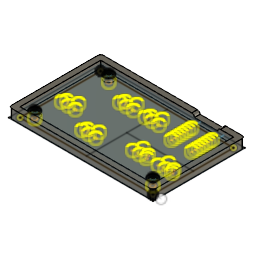
tetriopadv2_assembly (Autodesk Fusion 360 archive; units mm, degrees)
design "tetrio.padv2"
Autodesk Fusion 360 part; units mm, degrees
sketch "Sketch1" plane through (0, 0, -0.05) normal (0, 0, -1) x (1, 0, 0)
  line L0 (69.1388, 132.6388) -> (69.1388, 72.5424)
  line L1 (69.1388, 72.5424) -> (168.3004, 72.5424)
  line L2 (168.3004, 72.5424) -> (168.3004, 132.6388)
  line L3 (168.3004, 132.6388) -> (69.1388, 132.6388)
  circle A0 centre (75.184, 127.762) radius 1.5875
  circle A1 centre (162.6616, 127.1016) radius 1.5875
  circle A2 centre (105.5624, 117.7544) radius 1.9875
  circle A3 centre (100.4824, 117.7544) radius 0.8374
  circle A4 centre (110.6424, 117.7544) radius 0.8374
  circle A5 centre (101.7524, 115.2144) radius 0.7374
  circle A6 centre (137.5664, 111.8616) radius 1.9875
  circle A7 centre (156.6164, 111.8616) radius 1.9875
  circle A8 centre (108.1024, 112.6744) radius 0.7374
  circle A9 centre (132.4864, 111.8616) radius 0.8374
  circle A10 centre (142.6464, 111.8616) radius 0.8374
  circle A11 centre (151.5364, 111.8616) radius 0.8374
  circle A12 centre (161.6964, 111.8616) radius 0.8374
  circle A13 centre (141.3764, 109.3216) radius 0.7374
  circle A14 centre (160.4264, 109.3216) radius 0.7374
  circle A15 centre (79.5528, 106.9848) radius 1.9875
  circle A16 centre (74.4728, 106.9848) radius 0.8374
  circle A17 centre (84.6328, 106.9848) radius 0.8374
  circle A18 centre (135.0264, 106.7816) radius 0.7374
  circle A19 centre (154.0764, 106.7816) radius 0.7374
  circle A20 centre (75.7428, 104.4448) radius 0.7374
  circle A21 centre (82.0928, 101.9048) radius 0.7374
  circle A22 centre (140.0556, 90.7861) radius 0.4319
  circle A23 centre (155.2956, 90.7861) radius 0.4319
  circle A24 centre (140.0556, 88.2461) radius 0.4319
  circle A25 centre (155.2956, 88.2461) radius 0.4319
  circle A26 centre (101.8032, 85.8012) radius 1.9875
  circle A27 centre (120.8532, 85.8012) radius 1.9875
  circle A28 centre (96.7232, 85.8012) radius 0.8374
  circle A29 centre (106.8832, 85.8012) radius 0.8374
  circle A30 centre (115.7732, 85.8012) radius 0.8374
  circle A31 centre (125.9332, 85.8012) radius 0.8374
  circle A32 centre (140.0556, 85.7061) radius 0.4319
  circle A33 centre (155.2956, 85.7061) radius 0.4319
  circle A34 centre (97.9932, 83.2612) radius 0.7374
  circle A35 centre (117.0432, 83.2612) radius 0.7374
  circle A36 centre (140.0556, 83.1661) radius 0.4319
  circle A37 centre (155.2956, 83.1661) radius 0.4319
  circle A38 centre (104.3432, 80.7212) radius 0.7374
  circle A39 centre (123.3932, 80.7212) radius 0.7374
  circle A40 centre (140.0556, 80.6261) radius 0.4319
  circle A41 centre (155.2956, 80.6261) radius 0.4319
  circle A42 centre (140.0556, 78.0861) radius 0.4319
  circle A43 centre (155.2956, 78.0861) radius 0.4319
  circle A44 centre (79.2988, 76.6064) radius 1.5875
  circle A45 centre (140.0556, 75.5461) radius 0.4319
  circle A46 centre (155.2956, 75.5461) radius 0.4319
  circle A47 centre (75.184, 127.762) radius 1.5875
  circle A48 centre (79.2988, 76.6064) radius 1.5875
  circle A49 centre (162.6616, 127.1016) radius 1.5875
  circle A50 centre (162.6616, 127.1016) radius 3.5
  circle A51 centre (79.2988, 76.6064) radius 3.5
  circle A52 centre (75.184, 127.762) radius 3.5
  dimension "d1" = 7
  dimension "d2" = 7
  dimension "d3" = 7
  constraint concentric A0 A47
  constraint concentric A44 A48
  constraint concentric A1 A49
  constraint concentric A49 A50
  constraint concentric A48 A51
  constraint concentric A47 A52
  measures "d1" diameter of A50
  measures "d2" diameter of A51
  measures "d3" diameter of A52
extrude "Extrude1" add sketch "Sketch1" along normal blind 5 contours A50 | A51 | A52 makes body 1 at (72.8681, -125.1378, -3.3833) makes body 2 at (82.7944, -76.4319, -3.3833) makes body 3 at (165.4516, -129.2149, -3.3833)
sketch "Sketch2" plane through (0, 0, -0.05) normal (0, 0, -1) x (1, 0, 0)
sketch "Sketch3" plane through (0, 0, -5.05) normal (0, 0, -1) x (1, 0, 0)
  circle A0 centre (75.184, 127.762) radius 1.5875
  circle A1 centre (75.184, 127.762) radius 3.5
  line L0 (69.1388, 132.6388) -> (69.1388, 72.5424)
  line L1 (69.1388, 72.5424) -> (168.3004, 72.5424)
  line L2 (168.3004, 72.5424) -> (168.3004, 132.6388)
  line L3 (168.3004, 132.6388) -> (69.1388, 132.6388)
  circle A2 centre (75.184, 127.762) radius 1.5875
  circle A3 centre (162.6616, 127.1016) radius 1.5875
  circle A4 centre (105.5624, 117.7544) radius 1.9875
  circle A5 centre (100.4824, 117.7544) radius 0.8374
  circle A6 centre (110.6424, 117.7544) radius 0.8374
  circle A7 centre (101.7524, 115.2144) radius 0.7374
  circle A8 centre (137.5664, 111.8616) radius 1.9875
  circle A9 centre (156.6164, 111.8616) radius 1.9875
  circle A10 centre (108.1024, 112.6744) radius 0.7374
  circle A11 centre (132.4864, 111.8616) radius 0.8374
  circle A12 centre (142.6464, 111.8616) radius 0.8374
  circle A13 centre (151.5364, 111.8616) radius 0.8374
  circle A14 centre (161.6964, 111.8616) radius 0.8374
  circle A15 centre (141.3764, 109.3216) radius 0.7374
  circle A16 centre (160.4264, 109.3216) radius 0.7374
  circle A17 centre (79.5528, 106.9848) radius 1.9875
  circle A18 centre (74.4728, 106.9848) radius 0.8374
  circle A19 centre (84.6328, 106.9848) radius 0.8374
  circle A20 centre (135.0264, 106.7816) radius 0.7374
  circle A21 centre (154.0764, 106.7816) radius 0.7374
  circle A22 centre (75.7428, 104.4448) radius 0.7374
  circle A23 centre (82.0928, 101.9048) radius 0.7374
  circle A24 centre (140.0556, 90.7861) radius 0.4319
  circle A25 centre (155.2956, 90.7861) radius 0.4319
  circle A26 centre (140.0556, 88.2461) radius 0.4319
  circle A27 centre (155.2956, 88.2461) radius 0.4319
  circle A28 centre (101.8032, 85.8012) radius 1.9875
  circle A29 centre (120.8532, 85.8012) radius 1.9875
  circle A30 centre (96.7232, 85.8012) radius 0.8374
  circle A31 centre (106.8832, 85.8012) radius 0.8374
  circle A32 centre (115.7732, 85.8012) radius 0.8374
  circle A33 centre (125.9332, 85.8012) radius 0.8374
  circle A34 centre (140.0556, 85.7061) radius 0.4319
  circle A35 centre (155.2956, 85.7061) radius 0.4319
  circle A36 centre (97.9932, 83.2612) radius 0.7374
  circle A37 centre (117.0432, 83.2612) radius 0.7374
  circle A38 centre (140.0556, 83.1661) radius 0.4319
  circle A39 centre (155.2956, 83.1661) radius 0.4319
  circle A40 centre (104.3432, 80.7212) radius 0.7374
  circle A41 centre (123.3932, 80.7212) radius 0.7374
  circle A42 centre (140.0556, 80.6261) radius 0.4319
  circle A43 centre (155.2956, 80.6261) radius 0.4319
  circle A44 centre (140.0556, 78.0861) radius 0.4319
  circle A45 centre (155.2956, 78.0861) radius 0.4319
  circle A46 centre (79.2988, 76.6064) radius 1.5875
  circle A47 centre (140.0556, 75.5461) radius 0.4319
  circle A48 centre (155.2956, 75.5461) radius 0.4319
  line L4 (118.7196, 132.6388) -> (118.7196, 72.5424)
  line L5 (118.7196, 102.5906) -> (168.3004, 102.5906)
  line L6 (69.1388, 72.5424) -> (64.8962, 68.2998)
  line L7 (168.3004, 132.6388) -> (172.543, 136.8814)
  line L8 (168.3004, 132.6388) -> (174.3004, 132.6388) construction
  line L9 (64.8962, 68.2998) -> (172.543, 68.2998)
  line L10 (172.543, 68.2998) -> (172.543, 136.8814)
  line L11 (172.543, 136.8814) -> (64.8962, 136.8814)
  line L12 (64.8962, 136.8814) -> (64.8962, 68.2998)
  line L13 (69.1388, 72.5424) -> (168.3004, 72.5424)
  line L14 (168.3004, 72.5424) -> (168.3004, 132.6388)
  line L15 (168.3004, 132.6388) -> (69.1388, 132.6388)
  line L16 (69.1388, 132.6388) -> (69.1388, 72.5424)
  line L17 (139.1248, 68.2998) -> (139.1248, 72.5424)
  line L18 (156.4875, 72.5424) -> (156.4875, 68.2998)
  dimension "d6" = 6
  dimension "d7" = 45
  dimension "d8" = 45
  dimension "d9" = 6
  constraint midpoint L3 L4.start
  constraint midpoint L1 L4.end
  constraint midpoint L4 L5.start
  constraint midpoint L2 L5.end
  constraint coincident L0.end L1.start
  constraint horizontal L8
  constraint coincident L2.end L3.start
  constraint horizontal L9
  constraint vertical L10
  constraint horizontal L11
  constraint vertical L12
  constraint horizontal L13
  constraint vertical L14
  constraint horizontal L15
  constraint vertical L16
  constraint coincident L9 L17.start
  constraint coincident L13 L17.end
  constraint perpendicular L13 L17
  constraint coincident L13 L18.start
  constraint coincident L9 L18.end
  constraint perpendicular L9 L18
  measures "d6" distance of L0.end L6.end
  measures "d7" angle of L5 L6
  measures "d8" angle of L7 L8
  measures "d9" distance of L2.end L7.end
extrude "Extrude2" add sketch "Sketch3" against normal blind 7 separate body contours L0 L3 L6 L7 L11 L12 L15 L16 | L1 L6 L9 L13 L17 | L1 L2 L7 L9 L10 L13 L14 L18 makes body 4
sketch "Sketch4" plane through (0, 0, -5.05) normal (0, 0, -1) x (1, 0, 0)
  line L0 (168.3004, 132.6388) -> (69.1388, 132.6388)
  line L1 (69.1388, 132.6388) -> (69.1388, 72.5424)
  line L2 (69.1388, 72.5424) -> (168.3004, 72.5424)
  line L3 (168.3004, 72.5424) -> (168.3004, 132.6388)
  point P0 (69.1388, 72.5424)
  point P1 (168.3004, 132.6388)
  constraint horizontal L0
  constraint vertical L1
  constraint horizontal L2
  constraint vertical L3
  constraint coincident P0 L1.end
  constraint coincident P1 L0.start
extrude "Extrude3" add sketch "Sketch4" sketch "Sketch3" against normal blind 2 of sketch 2 contours A3 bodies 1 2 3 4
extrude "Extrude4" add sketch "Sketch3" against normal blind 2 contours L1 L9 L13 L17 L18 bodies 1
extrude "Extrude5" cut sketch "Sketch1" along normal mid plane 200 contours A0 A47 | A1 A49 | A44 A48 bodies 1
fillet "Fillet1" radius 2 2 edges at (156.4875, -70.4211, 1.95) (139.1248, -70.4211, 1.95) on bodies 1
fillet "Fillet2" radius 2 4 edges at (172.543, -68.2998, -1.55) (172.543, -136.8814, -1.55) (64.8962, -136.8814, -1.55) (64.8962, -68.2998, -1.55) on bodies 1
extrude "Extrude6" add sketch "Sketch3" against normal blind 5 contours L1 L9 L13 L17 L18 bodies 1
